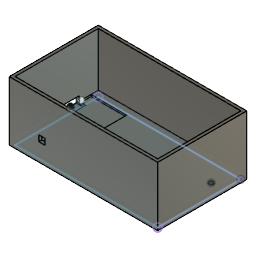
Enclosure (Autodesk Fusion 360 design; units mm, degrees)
part number: 2026-03-10-09-29-25-789
Autodesk Fusion 360 part; units mm, degrees
sketch "Sketch1" plane through (0, 0, 0) normal (0, 0, 1) x (1, 0, 0)
  line L0 (-40, 50) -> (210, 50)
  line L1 (210, 50) -> (210, -100)
  line L2 (210, -100) -> (-40, -100)
  line L3 (-40, -100) -> (-40, 50)
  line L4 (-35, 45) -> (205, 45)
  line L5 (205, 45) -> (205, -95)
  line L6 (205, -95) -> (-35, -95)
  line L7 (-35, -95) -> (-35, 45)
  dimension "d1" = 250
  dimension "d2" = 150
  dimension "d3" = 5
  dimension "d4" = 5
  dimension "d5" = 5
  dimension "d6" = 5
  constraint horizontal L0
  constraint vertical L1
  constraint horizontal L2
  constraint vertical L3
  constraint horizontal L4
  constraint vertical L5
  constraint horizontal L6
  constraint vertical L7
  measures "d1" distance of L0.start L0.end
  measures "d2" distance of L0 L2
  measures "d3" distance of L0 L4
  measures "d4" distance of L3 L7
  measures "d5" distance of L2 L6
  measures "d6" distance of L1 L5
sketch "Sketch2" plane through (0, 0, 0) normal (0, 0, 1) x (1, 0, 0)
  circle A0 centre (185, 15) radius 3.5
  line L0 (205, 45) -> (205, -95)
  line L1 (-35, 45) -> (205, 45)
  dimension "d7" = 7
  dimension "d8" = 20
  dimension "d9" = 30
  dimension "d12" = 20
  measures "d7" diameter of A0
  measures "d8" distance of A0.centre L0
  measures "d9" distance of A0.centre L1
  measures "d12" distance of A0.centre L0
sketch "Sketch3" plane through (0, 0, 0) normal (0, 0, 1) x (1, 0, 0)
extrude "Extrude1" add sketch "Sketch1" along normal blind 100
sketch "Sketch4" plane through (0, 0, 0) normal (0, 1, 0) x (1, 0, 0)
sketch "Sketch5" plane through (0, 0, 0) normal (0, 0, 1) x (1, 0, 0)
  line L0 (-35, 45) -> (205, 45)
  line L1 (205, 45) -> (205, -95)
  line L2 (205, -95) -> (-35, -95)
  line L3 (-35, -95) -> (-35, 45)
  constraint horizontal L0
  constraint vertical L1
  constraint horizontal L2
  constraint vertical L3
extrude "Extrude2" add sketch "Sketch5" along normal blind 10
sketch "Sketch6" plane through (0, 0, 10) normal (0, 0, 1) x (-1, 0, 0)
  line L0 (35, 95) -> (-205, 95)
  line L1 (-205, 95) -> (-205, -45)
  line L2 (-205, -45) -> (35, -45)
  line L3 (35, -45) -> (35, 95)
  circle A0 centre (-185, -15) radius 3.6056
extrude "Extrude3" cut sketch "Sketch6" against normal blind 10 contours A0
sketch "Sketch7" plane through (0, 0, 0) normal (0, 0, 1) x (1, 0, 0)
  line L0 (-20, -50) -> (5.5, -50)
  line L1 (5.5, -50) -> (5.5, -35.9)
  line L2 (5.5, -35.9) -> (-20, -35.9)
  line L3 (-20, -35.9) -> (-20, -50)
  line L4 (210, -100) -> (-40, -100)
  dimension "d20" = 25.5
  dimension "d21" = 14.1
  dimension "d22" = 50
  constraint horizontal L0
  constraint vertical L1
  constraint horizontal L2
  constraint vertical L3
  measures "d20" distance of L0.start L0.end
  measures "d21" distance of L0.start L2.end
  measures "d22" distance of L0 L4
extrude "Extrude4" cut sketch "Sketch7" along normal blind 10
sketch "Sketch8" plane through (0, 0, 10) normal (0, 0, 1) x (-1, 0, 0)
  line L0 (20, 35.9) -> (-5.5, 35.9)
  line L1 (-5.5, 35.9) -> (-5.5, 50)
  line L2 (-5.5, 50) -> (20, 50)
  line L3 (20, 50) -> (20, 35.9)
  circle A0 centre (-185, -15) radius 3.6056
  line L4 (35, 95) -> (-205, 95)
  line L5 (-205, 95) -> (-205, -45)
  line L6 (-205, -45) -> (35, -45)
  line L7 (35, -45) -> (35, 95)
  line L8 (22.8, 30.9) -> (-7.2, 30.9)
  line L9 (-7.2, 30.9) -> (-7.2, 59.9)
  line L10 (-7.2, 59.9) -> (22.8, 59.9)
  line L11 (22.8, 59.9) -> (22.8, 30.9)
  dimension "d25" = 30
  dimension "d26" = 29
  dimension "d27" = 5
  dimension "d28" = 1.7
  dimension "d29" = 29
  constraint horizontal L8
  constraint vertical L9
  constraint horizontal L10
  constraint vertical L11
  measures "d25" distance of L8.start L8.end
  measures "d26" distance of L8.start L10.end
  measures "d27" distance of L0 L8
  measures "d28" distance of L1 L9
  measures "d29" distance of L8.start L10.end
extrude "Extrude5" cut sketch "Sketch8" against normal blind 7 contours L8 L9 L10 L11
sketch "Sketch9" plane through (0, 0, 10) normal (0, 0, 1) x (-1, 0, 0)
  line L0 (-7.2, 30.9) -> (-7.2, 59.9)
  line L1 (-7.2, 59.9) -> (22.8, 59.9)
  line L2 (22.8, 59.9) -> (22.8, 30.9)
  line L3 (22.8, 30.9) -> (-7.2, 30.9)
  circle A0 centre (-185, -15) radius 3.6056
  line L4 (35, 95) -> (-205, 95)
  line L5 (-205, 95) -> (-205, -45)
  line L6 (-205, -45) -> (35, -45)
  line L7 (35, -45) -> (35, 95)
sketch "Sketch10" plane through (0, 0, 10) normal (0, 0, 1) x (-1, 0, 0)
sketch "Sketch11" plane through (0, 0, 10) normal (0, 0, 1) x (-1, 0, 0)
  line L0 (34.9, -32.7882) -> (-25.2, -32.7882)
  line L1 (-25.2, -32.7882) -> (-25.2, 17.7118)
  line L2 (-25.2, 17.7118) -> (34.9, 17.7118)
  line L3 (34.9, 17.7118) -> (34.9, -32.7882)
  line L4 (35.6, -7.5382) -> (29.9, -7.5382)
  line L5 (29.9, -7.5382) -> (29.9, -15.5382)
  line L6 (29.9, -15.5382) -> (35.6, -15.5382)
  line L7 (35.6, -15.5382) -> (35.6, -7.5382)
  line L8 (35, 95) -> (35, -45)
  dimension "d38" = 60.1
  dimension "d39" = 50.5
  dimension "d40" = 5.7
  dimension "d41" = 8
  dimension "d42" = 55.1
  dimension "d43" = 0.1
  constraint horizontal L0
  constraint vertical L1
  constraint horizontal L2
  constraint vertical L3
  constraint horizontal L4
  constraint vertical L5
  constraint horizontal L6
  constraint vertical L7
  measures "d38" distance of L0.start L0.end
  measures "d39" distance of L0.start L2.end
  measures "d40" distance of L4.start L4.end
  measures "d41" distance of L4.start L6.end
  measures "d42" distance of L1 L5
  measures "d43" distance of L3 L8
sketch "Sketch12" plane through (0, 0, 0) normal (1, 0, 0) x (0, 1, 0)
sketch "Sketch13" plane through (-40, 0, 0) normal (-1, 0, 0) x (0, -1, 0)
  line L0 (-50, 0) -> (100, 0)
  line L1 (100, 0) -> (100, 100)
  line L2 (100, 100) -> (-50, 100)
  line L3 (-50, 100) -> (-50, 0)
  line L4 (-19.2882, 18) -> (-4.2882, 18)
  line L5 (-4.2882, 18) -> (-4.2882, 3)
  line L6 (-4.2882, 3) -> (-19.2882, 3)
  line L7 (-19.2882, 3) -> (-19.2882, 18)
  line L8 (-15.5382, 10) -> (-7.5382, 10)
  dimension "d44" = 15
  dimension "d45" = 15
  dimension "d46" = 8
  dimension "d47" = 3.75
  constraint horizontal L4
  constraint vertical L5
  constraint horizontal L6
  constraint vertical L7
  measures "d44" distance of L4.start L4.end
  measures "d45" distance of L4.start L6.end
  measures "d46" distance of L4 L8
  measures "d47" distance of L7 L8.start
extrude "Extrude6" cut sketch "Sketch13" against normal blind 13 contours L4 L5 L6 L7
extrude "Extrude7" cut sketch "Sketch11" against normal blind 3 contours L0 L1 L2 L3 L4 L5 L6
sketch "Sketch14" plane through (0, 0, 0) normal (0, 0, 1) x (1, 0, 0)
sketch "Sketch15" plane through (0, 0, 0) normal (0, 0, 1) x (1, 0, 0)
sketch "Sketch16" plane through (0, -100, 0) normal (0, -1, 0) x (1, 0, 0)
  line L0 (-40, 0) -> (210, 0)
  line L1 (210, 0) -> (210, 100)
  line L2 (210, 100) -> (-40, 100)
  line L3 (-40, 100) -> (-40, 0)
  line L4 (10, 40) -> (20.2, 40)
  line L5 (20.2, 40) -> (20.2, 30)
  line L6 (20.2, 30) -> (10, 30)
  line L7 (10, 30) -> (10, 40)
  line L8 (205, 0) -> (-35, 0)
  dimension "d52" = 10.2
  dimension "d53" = 10
  dimension "d54" = 30
  dimension "d55" = 50
  constraint horizontal L4
  constraint vertical L5
  constraint horizontal L6
  constraint vertical L7
  measures "d52" distance of L4.start L4.end
  measures "d53" distance of L4.start L6.end
  measures "d54" distance of L6 L8
  measures "d55" distance of L3 L7
extrude "Extrude8" cut sketch "Sketch16" against normal blind 10 contours L4 L5 L6 L7
sketch "Sketch17" plane through (-40, 0, 0) normal (-1, 0, 0) x (0, -1, 0)
  line L0 (-4.2882, 18) -> (-4.2882, 3)
  line L1 (-4.2882, 3) -> (-19.2882, 3)
  line L2 (-19.2882, 3) -> (-19.2882, 18)
  line L3 (-19.2882, 18) -> (-4.2882, 18)
  line L4 (-50, 0) -> (100, 0)
  line L5 (100, 0) -> (100, 100)
  line L6 (100, 100) -> (-50, 100)
  line L7 (-50, 100) -> (-50, 0)
  line L8 (-19.2882, 18) -> (-4.2882, 18)
  line L9 (-4.2882, 18) -> (-4.2882, 3)
  line L10 (-4.2882, 3) -> (-19.2882, 3)
  line L11 (-19.2882, 3) -> (-19.2882, 18)
  constraint horizontal L8
  constraint vertical L9
  constraint horizontal L10
  constraint vertical L11
  constraint coincident L0.end L1.start
  constraint coincident L2.end L3.start
extrude "Extrude9" add sketch "Sketch17" against normal blind 13 contours L0 L1 L2 L3 L8 L9 L10 L11
sketch "Sketch18" plane through (0, 0, 10) normal (0, 0, 1) x (-1, 0, 0)
  line L0 (26.9999, 2.0114) -> (35, 2.0114)
  line L1 (35, 2.0114) -> (35, -15.984)
  line L2 (35, -15.984) -> (26.9999, -15.984)
  line L3 (26.9999, -15.984) -> (26.9999, 2.0114)
  constraint horizontal L0
  constraint vertical L1
  constraint horizontal L2
  constraint vertical L3
extrude "Extrude10" cut 1 faces at (-32.3333, 14.2882, 18) along direction (0, 0, -1) blind 11
extrude "Extrude11" cut sketch "Sketch18" against normal blind 4
sketch "Sketch19" plane through (-35, 0, 0) normal (1, 0, 0) x (0, 1, 0)
  line L0 (15.984, 7) -> (19.2882, 7)
  line L1 (19.2882, 7) -> (19.2882, 10)
  line L2 (19.2882, 10) -> (45, 10)
  line L3 (45, 10) -> (45, 100)
  line L4 (45, 100) -> (-95, 100)
  line L5 (-95, 100) -> (-95, 10)
  line L6 (-95, 10) -> (-2.0114, 10)
  line L7 (-2.0114, 10) -> (-2.0114, 6)
  line L8 (-2.0114, 6) -> (15.984, 6)
  line L9 (15.984, 6) -> (15.984, 7)
  line L10 (-2.0114, 10) -> (15.984, 10)
  line L11 (-2.0114, 7) -> (-2.0114, 10)
  constraint horizontal L10
  constraint vertical L11
  constraint coincident L6.end L7.start
sketch "Sketch20" plane through (-35, 0, 0) normal (1, 0, 0) x (0, 1, 0)
sketch "Sketch21" plane through (-35, 0, 0) normal (1, 0, 0) x (0, 1, 0)
  line L0 (-2, 10) -> (16, 10)
  line L1 (16, 10) -> (16, 7)
  line L2 (16, 7) -> (-2, 7)
  line L3 (-2, 7) -> (-2, 10)
  constraint horizontal L0
  constraint vertical L1
  constraint horizontal L2
  constraint vertical L3
sketch "Sketch22" plane through (-40, 0, 0) normal (-1, 0, 0) x (0, -1, 0)
  line L0 (-50, 0) -> (100, 0)
  line L1 (100, 0) -> (100, 100)
  line L2 (100, 100) -> (-50, 100)
  line L3 (-50, 100) -> (-50, 0)
  line L4 (-16, 10) -> (2, 10)
  line L5 (2, 10) -> (2, 7)
  line L6 (2, 7) -> (-16, 7)
  line L7 (-16, 7) -> (-16, 10)
  constraint horizontal L4
  constraint vertical L5
  constraint horizontal L6
  constraint vertical L7
extrude "Extrude12" cut sketch "Sketch22" against normal blind 6 contours L4 L5 L6 L7
sketch "Sketch23" plane through (-35, 0, 0) normal (1, 0, 0) x (0, 1, 0)
sketch "Sketch24" plane through (-40, 0, 0) normal (-1, 0, 0) x (0, -1, 0)
  line L0 (2, 10) -> (2, 7)
  line L1 (2, 7) -> (-16, 7)
  line L2 (-16, 7) -> (-16, 10)
  line L3 (-16, 10) -> (2, 10)
  line L4 (-50, 0) -> (100, 0)
  line L5 (100, 0) -> (100, 100)
  line L6 (100, 100) -> (-50, 100)
  line L7 (-50, 100) -> (-50, 0)
  line L8 (-16, 14) -> (2, 14)
  line L9 (2, 14) -> (2, 6)
  line L10 (2, 6) -> (-16, 6)
  line L11 (-16, 6) -> (-16, 14)
  constraint horizontal L8
  constraint vertical L9
  constraint horizontal L10
  constraint vertical L11
extrude "Extrude13" cut sketch "Sketch24" against normal blind 58 contours L3 L8 L9 L11
sketch "Sketch25" plane through (-35, 0, 0) normal (1, 0, 0) x (0, 1, 0)
extrude "Extrude14" add sketch "Sketch21" against normal blind 5
sketch "Sketch26" plane through (-35, 0, 0) normal (1, 0, 0) x (0, 1, 0)
  line L0 (16, 14) -> (-2, 14)
  line L1 (-2, 14) -> (-2, 10)
  line L2 (-2, 10) -> (16, 10)
  line L3 (16, 10) -> (16, 14)
  constraint horizontal L0
  constraint vertical L1
  constraint horizontal L2
  constraint vertical L3
extrude "Extrude15" add sketch "Sketch26" against normal blind 5
sketch "Sketch27" plane through (0, 0, 10) normal (0, 0, 1) x (-1, 0, 0)
  line L0 (27, 12) -> (35, 12)
  line L1 (35, 12) -> (35, 2)
  line L2 (35, 2) -> (27, 2)
  line L3 (27, 2) -> (27, 12)
  constraint horizontal L0
  constraint vertical L1
  constraint horizontal L2
  constraint vertical L3
extrude "Extrude16" cut sketch "Sketch27" against normal blind 4
sketch "Sketch28" plane through (0, 0, 10) normal (0, 0, 1) x (-1, 0, 0)
sketch "Sketch29" plane through (0, 0, 10) normal (0, 0, 1) x (-1, 0, 0)
sketch "Sketch30" plane through (0, 0, 0) normal (1, 0, 0) x (0, 1, 0)
sketch "Sketch31" plane through (-40, 0, 0) normal (-1, 0, 0) x (0, -1, 0)
  line L0 (-50, 0) -> (100, 0)
  line L1 (100, 0) -> (100, 100)
  line L2 (100, 100) -> (-50, 100)
  line L3 (-50, 100) -> (-50, 0)
  line L4 (-12.7294, 18) -> (11.2444, 18)
  line L5 (11.2444, 18) -> (11.2444, 5)
  line L6 (11.2444, 5) -> (-12.7294, 5)
  line L7 (-12.7294, 5) -> (-12.7294, 18)
  constraint horizontal L4
  constraint vertical L5
  constraint horizontal L6
  constraint vertical L7
extrude "Extrude17" cut sketch "Sketch31" against normal blind 13 contours L4 L5 L6 L7
